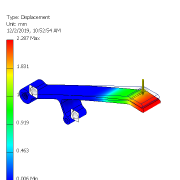
# Autodesk Inventor part: part
Saved by Autodesk Inventor 2020.1 (Build 241239000, 239)
## iProperties
Created: 2019-11-25
Part Number: part
Material: Aluminum 6061
Document SubType Name: Modeling
Designer: Rafi
Density: 2.7 g/cm^3
Appearance: Aluminum - Flat
Author: Rafi
Autodesk Inventor part; units mm, degrees
ref_plane "YZ Plane" through (0, 0, 0) normal (1, 0, 0) x (0, 1, 0)
ref_plane "XZ Plane" through (0, 0, 0) normal (0, 1, 0) x (-1, 0, 0)
ref_plane "XY Plane" through (0, 0, 0) normal (0, 0, 1) x (1, 0, 0)
sketch "Sketch1" plane through (0, 0, 0) normal (0, 0, 1) x (1, 0, 0)
  line L0 (0, 0) -> (62, 30) construction
  line L1 (62, 30) -> (70, 30) construction
  line L2 (20.2572, 9.8019) -> (25, 0) construction
  circle A0 centre (0, 0) radius 1.5
  circle A1 centre (25, 0) radius 1
  arc A2 (2.5837, 2.3611) -> (3.4548, 0.5608) centre (0, 0) ccw
  arc A3 (23.7065, 1.5254) -> (24.6066, 1.9609) centre (25, 0) ccw
  line L3 (3.4548, 0.5608) -> (20.2426, 8.6839)
  line L4 (20.2426, 8.6839) -> (23.7065, 1.5254)
  line L5 (24.6066, 1.9609) -> (21.1428, 9.1195)
  line L6 (21.1428, 9.1195) -> (62.2292, 29)
  line L7 (62.2292, 29) -> (70, 29)
  arc A4 (70, 29) -> (70, 31) centre (70, 30) ccw
  line L8 (70, 31) -> (61.7708, 31)
  line L9 (61.7708, 31) -> (2.5837, 2.3611)
  dimension "d0" = 25
  dimension "d1" = 70
  dimension "d2" = 8
  dimension "d3" = 30
  dimension "d4" = 3
  dimension "d5" = 2
  dimension "d6" = 7
  dimension "d7" = 4
  dimension "d8" = 1
  dimension "d9" = 1
  dimension "d10" = 1
  dimension "d11" = 1
  dimension "d12" = 0.5
  dimension "d13" = 0.5
  constraints: 20 end point, 6 parallel, 6 point on circle, 5 centre point, 4 coincident, 2 horizontal, 2 tangent, 1 collinear, 1 horizontal alignment, 1 perpendicular, 1 point on line, 1 vertical alignment
  measures "d0" distance of L2.end L0.start
  measures "d1" horizontal distance of L1.end L0.start
  measures "d2" distance of L1.end L0.end
  measures "d3" distance from line of L2.end L1
  measures "d4" diameter of A0
  measures "d5" diameter of A1
  measures "d6" diameter of A2
  measures "d7" diameter of A3
  measures "d8" distance between parallel lines of L0 L3
  measures "d9" distance between parallel lines of L0 L9
  measures "d10" distance between parallel lines of L1 L8
  measures "d11" distance between parallel lines of L1 L7
  measures "d12" distance between parallel lines of L2 L4
  measures "d13" distance between parallel lines of L2 L5
extrude "Extrusion1" add sketch "Sketch1" along normal mid plane 10
fillet "Fillet1" radius 2 8 edges at (3.4548, 0.5608, 0) (2.5837, 2.3611, 0) (21.1428, 9.1195, 0) (20.2426, 8.6839, 0) (62.2292, 29, 0) (61.7708, 31, 0) (24.6066, 1.9609, 0) (23.7065, 1.5254, 0)
body "Solid1"
